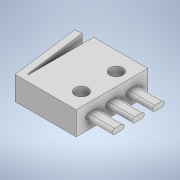
# Autodesk Inventor part: micro_switch_1
Saved by Autodesk Inventor 2020 (Build 240168000, 168)
## iProperties
Created: 2019-08-05
Part Number: micro_switch_1
Material: Generic
Document SubType Name: Modeling
Designer: psrob
Density: 1 g/cm^3
Appearance: Default
Author: psrob
Autodesk Inventor part; units mm, degrees
ref_plane "YZ Plane" through (0, 0, 0) normal (1, 0, 0) x (0, 1, 0)
ref_plane "XZ Plane" through (0, 0, 0) normal (0, 1, 0) x (-1, 0, 0)
ref_plane "XY Plane" through (0, 0, 0) normal (0, 0, 1) x (1, 0, 0)
sketch "Sketch1" plane through (0, 0, 0) normal (0, 1, 0) x (-1, 0, 0)
  line L0 (0, 0) -> (6.2, 0)
  line L1 (6.2, 0) -> (6.2, -8.2)
  line L2 (6.2, -8.2) -> (0, -8.2)
  line L3 (0, -8.2) -> (0, 0)
  dimension "d0" = 8.2
  dimension "d1" = 6.2
  constraints: 8 end point, 2 parallel, 1 horizontal, 1 perpendicular
  measures "d0" distance of L0.end L1.end
  measures "d1" distance of L1.end L2.end
extrude "Extrusion1" add sketch "Sketch1" along normal blind 2.7
sketch "Sketch2" plane through (0, 2.7, 0) normal (0, 1, 0) x (1, 0, 0)
  line L0 (-6.2, 8.2) -> (-6.2, 0) projected
  line L1 (-6.2, 0) -> (0, 0) projected
  line L2 (0, 0) -> (0, 8.2) projected
  line L3 (0, 8.2) -> (-6.2, 8.2) projected
  line L4 (-6.2, 8.2) -> (-6.2, 0) projected
  line L5 (-6.2, 0) -> (-7.2442, 7.9316)
  line L6 (-7.2442, 7.9316) -> (-8.0374, 7.8271)
  line L7 (-8.0374, 7.8271) -> (-7.0069, 0)
  line L8 (-6.2, 0) -> (-7.0069, 0)
  dimension "d4" = 8
  dimension "d5" = 7.5
  dimension "d6" = 0.8
  constraints: 8 end point, 2 perpendicular, 1 horizontal, 1 parallel
  measures "d4" distance of L0.end L5.end
  measures "d5" angle of L0 L5
  measures "d6" distance of L5.end L6.end
extrude "Extrusion2" add sketch "Sketch2" against normal up to surface (2.7 mm away) contours L8 L7 L6 L5
sketch "Sketch3" plane through (0, 0, 0) normal (0, -1, 0) x (1, 0, 0)
  line L0 (-6.2, -8.2) -> (-6.2, 0) projected
  line L1 (0, -8.2) -> (-6.2, -8.2) projected
  line L2 (0, 0) -> (0, -8.2) projected
  line L3 (-6.2, 0) -> (0, 0) projected
  line L4 (-7.0069, 0) -> (-8.0374, -7.8271) projected
  line L5 (-8.0374, -7.8271) -> (-7.2442, -7.9316) projected
  line L6 (-7.2442, -7.9316) -> (-6.2, 0) projected
  line L7 (-6.2, 0) -> (-7.0069, 0) projected
  line L8 (-6.2, 0) -> (0, 0) projected
  circle A0 centre (-6.2, 0) radius 0.75
  point P0 (-6.2979, -0.7436)
  point P1 (-6.2, -0.75)
  dimension "d9" = 1.5
  constraints: 1 centre point, 1 coincident
  measures "d9" diameter of A0
extrude "Extrusion3" add sketch "Sketch3" against normal up to surface (2.7 mm away) contours A0 L6 L0
sketch "Sketch4" plane through (0, 2.7, 0) normal (0, 1, 0) x (1, 0, 0)
  line L0 (-6.2, 8.2) -> (-6.2, 0.75) projected
  arc A0 (-6.2, 0.75) -> (-6.2979, 0.7436) centre (-6.2, 0) ccw projected
  line L1 (-6.2979, 0.7436) -> (-7.2442, 7.9316) projected
  line L2 (-7.2442, 7.9316) -> (-8.0374, 7.8271) projected
  line L3 (-8.0374, 7.8271) -> (-7.0069, 0) projected
  line L4 (-7.0069, 0) -> (0, 0) projected
  line L5 (0, 0) -> (0, 8.2) projected
  line L6 (0, 8.2) -> (-6.2, 8.2) projected
  line L7 (0, 0) -> (0, 8.2) projected
  line L8 (0, 4.1) -> (-1.5, 4.1)
  line L9 (-1.5, 4.1) -> (-1.5, 6.1)
  line L10 (-1.5, 4.1) -> (-1.5, 2.1)
  circle A1 centre (-1.5, 2.1) radius 0.75
  circle A2 centre (-1.5, 6.1) radius 0.75
  dimension "d12" = 1.5
  dimension "d13" = 2
  dimension "d14" = 2
  dimension "d15" = 1.5
  dimension "d16" = 1.5
  constraints: 6 end point, 2 centre point, 2 coincident, 2 vertical, 1 horizontal, 1 midpoint
  measures "d12" distance of L8.start L8.end
  measures "d13" distance of L8.end L9.end
  measures "d14" distance of L8.end L10.end
  measures "d15" diameter of A1
  measures "d16" diameter of A2
extrude "Extrusion4" cut sketch "Sketch4" against normal blind 2.7 contours A1 | A2
sketch "Sketch5" plane through (0, 0, 0) normal (1, 0, 0) x (0, 0, -1)
  line L0 (0, 0) -> (8.2, 0) projected
  line L1 (8.2, 0) -> (8.2, 2.7) projected
  line L2 (0, 2.7) -> (8.2, 2.7) projected
  line L3 (0, 0) -> (0, 2.7) projected
  line L4 (0.7436, 2.7) -> (7.9316, 2.7) projected
  line L5 (4.1, 2.7) -> (4.1, 1.35)
  line L6 (7.9316, 0) -> (0.7436, 0) projected
  line L7 (3.7, 1.35) -> (4.5, 1.35) construction
  line L8 (3.7, 1.05) -> (4.5, 1.05)
  line L9 (4.5, 1.65) -> (3.7, 1.65)
  arc A0 (3.7, 1.65) -> (3.7, 1.05) centre (3.7, 1.35) ccw
  arc A1 (4.5, 1.05) -> (4.5, 1.65) centre (4.5, 1.35) ccw
  line L10 (4.1, 1.35) -> (6.4, 1.35)
  line L11 (6, 1.35) -> (6.8, 1.35) construction
  line L12 (6, 1.05) -> (6.8, 1.05)
  line L13 (6.8, 1.65) -> (6, 1.65)
  arc A2 (6, 1.65) -> (6, 1.05) centre (6, 1.35) ccw
  arc A3 (6.8, 1.05) -> (6.8, 1.65) centre (6.8, 1.35) ccw
  line L14 (4.1, 1.35) -> (1.8, 1.35)
  line L15 (1.4, 1.35) -> (2.2, 1.35) construction
  line L16 (1.4, 1.05) -> (2.2, 1.05)
  line L17 (2.2, 1.65) -> (1.4, 1.65)
  arc A4 (1.4, 1.65) -> (1.4, 1.05) centre (1.4, 1.35) ccw
  arc A5 (2.2, 1.05) -> (2.2, 1.65) centre (2.2, 1.35) ccw
  dimension "d19" = 1.35
  dimension "d20" = 0.4
  dimension "d21" = 0.6
  dimension "d22" = 2.3
  dimension "d23" = 0.4
  dimension "d24" = 0.6
  dimension "d25" = 2.3
  dimension "d26" = 0.4
  dimension "d27" = 0.6
  constraints: 30 end point, 12 point on circle, 12 tangent, 6 centre point, 4 horizontal, 3 midpoint, 3 parallel, 2 point on line, 1 perpendicular
  measures "d19" distance of L5.start L5.end
  measures "d20" distance of L5.end L7.end
  measures "d21" diameter of A1
  measures "d22" distance of L5.end L10.end
  measures "d23" distance of L10.end L11.end
  measures "d24" diameter of A3
  measures "d25" distance of L5.end L14.end
  measures "d26" distance of L14.end L15.end
  measures "d27" diameter of A5
extrude "Extrusion5" add sketch "Sketch5" along normal blind 3 contours A2 L13 A3 L12 | A5 L16 A4 L17 | L9 A1 L10 L5 | L5 L14 A0 L9 | L10 A1 L8 A0 L14
body "Solid1"
